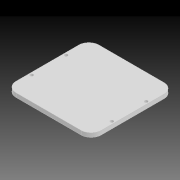
# Autodesk Inventor part: KB33-046-004-021 - Зажим точки доступа
Saved by Autodesk Inventor 2020 (Build 240168000, 168)
## iProperties
Created: 2021-08-18
Part Number: KB33-046-004-021 - Зажим точки доступа
Material: Типовые
Document SubType Name: Modeling
Designer: Петров Иван
Density: 1 g/cm^3
Appearance: По умолчанию
Mass: 27.1775 g
Surface Area: 150.009 cm^2
Volume: 27.1775 cm^3
Author: Петров Иван
Autodesk Inventor part; units mm, degrees
ref_plane "YZ Plane" through (0, 0, 0) normal (1, 0, 0) x (0, 1, 0)
ref_plane "XZ Plane" through (0, 0, 0) normal (0, 1, 0) x (-1, 0, 0)
ref_plane "XY Plane" through (0, 0, 0) normal (0, 0, 1) x (1, 0, 0)
sketch "Эскиз1" plane through (0, 0, 0) normal (0, 1, 0) x (-1, 0, 0)
  line L0 (42, 40) -> (42, 38)
  line L1 (-28.1339, -42) -> (-42.25, -42)
  line L2 (42, 40) -> (-42.25, 40)
  line L3 (-42.25, 40) -> (-42.25, -42)
  line L4 (-42.25, -42) -> (42, -42)
  line L5 (42, -42) -> (42, 40)
  circle A0 centre (39.5, -17) radius 1.5
  circle A1 centre (-39.75, -17) radius 1.5
  circle A2 centre (-39.75, 17) radius 1.5
  circle A3 centre (39.5, 17) radius 1.5
  point P0 (0, 0)
  point P1 (0, 0)
  constraints: 12 end point, 4 centre point, 2 parallel, 1 horizontal, 1 perpendicular
extrude "Выдавливание1" add sketch "Эскиз1" along normal blind 4
fillet "Сопряжение1" radius 10 4 edges at (42.25, 2, 40) (42.25, 2, -42) (-42, 2, -42) (-42, 2, 40)
